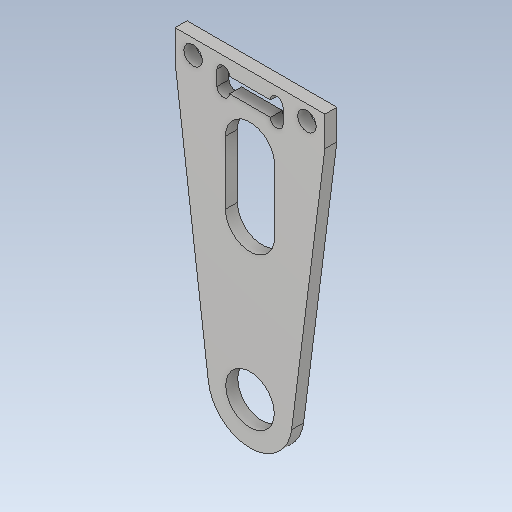
# Autodesk Inventor part: Leg_joint_slider_frame
Saved by Autodesk Inventor 2020.4 (Build 244396000, 396)
## iProperties
Part Number: Leg_joint_slider_frame
Material: アルミニウム 2014-T4
Document SubType Name: Modeling
Designer: Masato Kubotera
Density: 2.8 g/cm^3
Appearance: 滑らか - 淡い灰色
Mass: 4.69686 g
Surface Area: 22.2791 cm^2
Volume: 1.67745 cm^3
Description: A2017 T2
Author: Masato Kubotera
Autodesk Inventor part; units mm, degrees
ref_plane "YZ Plane" through (0, 0, 0) normal (1, 0, 0) x (0, 1, 0)
ref_plane "XZ Plane" through (0, 0, 0) normal (0, 1, 0) x (-1, 0, 0)
ref_plane "XY Plane" through (0, 0, 0) normal (0, 0, 1) x (1, 0, 0)
derived "Leg_joint_roll_basis.ipt"
sketch "スケッチ1" plane through (0, 0, 0) normal (0, 0, 1) x (1, 0, 0)
  circle A0 centre (0, 0) radius 11 construction
  line L0 (-13.5, -1) -> (13.5, -1) construction
  line L1 (13.5, -1) -> (13.5, -28) construction
  line L2 (13.5, -28) -> (-13.5, -28) construction
  line L3 (-13.5, -28) -> (-13.5, -1) construction
  line L4 (0, 18) -> (0, -18) construction
  circle A1 centre (0, -18) radius 7 construction
  line L5 (-12.5, 29.5) -> (-12.5, 24.5)
  line L6 (-12.5, 24.5) -> (-6.9433, -18.8892)
  line L7 (-12.5, 29.5) -> (12.5, 29.5)
  line L8 (12.5, 29.5) -> (12.5, 24.5)
  line L9 (12.5, 24.5) -> (6.9433, -18.8892)
  arc A2 (-6.9433, -18.8892) -> (6.9433, -18.8892) centre (0, -18) ccw
  circle A3 centre (-9.5, 27) radius 1.55
  circle A4 centre (9.5, 27) radius 1.55
  line L10 (-5.51, 27.01) -> (5.51, 27.01)
  line L11 (5.51, 27.01) -> (5.51, 24.49)
  line L12 (5.51, 24.49) -> (-5.51, 24.49)
  line L13 (-5.51, 24.49) -> (-5.51, 27.01)
  circle A5 centre (-4.46, 27.01) radius 1.05
  circle A6 centre (-4.46, 24.49) radius 1.05
  circle A7 centre (4.46, 27.01) radius 1.05
  circle A8 centre (4.46, 24.49) radius 1.05
  line L14 (5.5, 27) -> (-5.5, 27) construction
  line L15 (-5.5, 27) -> (-5.5, 24.5) construction
  line L16 (-5.5, 24.5) -> (5.5, 24.5) construction
  line L17 (5.5, 24.5) -> (5.5, 27) construction
  circle A9 centre (0, -18) radius 4.05
  circle A10 centre (0, 8.5) radius 1.35 construction
  circle A11 centre (-8.5, 0) radius 1.35 construction
  circle A12 centre (0, -8.5) radius 1.35 construction
  circle A13 centre (8.5, 0) radius 1.35 construction
  circle A14 centre (0, 0) radius 5.05 construction
  line L18 (-10.5671, 3.0556) -> (-5.7639, 19.6667) construction
  line L19 (5.7639, 19.6667) -> (10.5671, 3.0556) construction
  arc A15 (-10.5671, 3.0556) -> (10.5671, 3.0556) centre (0, 0) ccw construction
  arc A16 (5.7639, 19.6667) -> (-5.7639, 19.6667) centre (0, 18) ccw construction
  circle A17 centre (0, 18) radius 2.25 construction
  line L20 (-10.9105, 1.4) -> (-14.2125, 1.4) construction
  line L21 (-14.2125, 1.4) -> (-24.81, -5.5) construction
  line L22 (-24.81, -5.5) -> (-24.81, -23.5) construction
  line L23 (-24.81, -23.5) -> (-14.2125, -30.4) construction
  line L24 (-14.2125, -30.4) -> (14.2125, -30.4) construction
  line L25 (14.2125, -30.4) -> (24.81, -23.5) construction
  line L26 (24.81, -23.5) -> (24.81, -5.5) construction
  line L27 (24.81, -5.5) -> (14.2125, 1.4) construction
  line L28 (14.2125, 1.4) -> (10.9105, 1.4) construction
  arc A18 (-10.9105, 1.4) -> (10.9105, 1.4) centre (0, 0) ccw construction
  line L29 (-21.76, -10.49) -> (-19.74, -10.49) construction
  line L30 (-19.74, -10.49) -> (-19.74, -18.51) construction
  line L31 (-19.74, -18.51) -> (-21.76, -18.51) construction
  line L32 (-21.76, -18.51) -> (-21.76, -10.49) construction
  line L33 (-19.75, -10.5) -> (-21.75, -10.5) construction
  line L34 (-21.75, -10.5) -> (-21.75, -18.5) construction
  line L35 (-21.75, -18.5) -> (-19.75, -18.5) construction
  line L36 (-19.75, -18.5) -> (-19.75, -10.5) construction
  circle A19 centre (-21.76, -11.54) radius 1.05 construction
  circle A20 centre (-19.74, -11.54) radius 1.05 construction
  circle A21 centre (-19.74, -17.46) radius 1.05 construction
  circle A22 centre (-21.76, -17.46) radius 1.05 construction
  circle A23 centre (-13.5, -1) radius 2.4 construction
  line L37 (-24.81, -14.5) -> (-19.75, -14.5) construction
  circle A24 centre (-21.76, -11.54) radius 3.05 construction
  circle A25 centre (-13.5, -28) radius 2.4 construction
  line L38 (21.76, -10.49) -> (19.74, -10.49) construction
  line L39 (19.75, -10.5) -> (21.75, -10.5) construction
  circle A26 centre (19.74, -11.54) radius 1.05 construction
  circle A27 centre (21.76, -11.54) radius 1.05 construction
  circle A28 centre (21.76, -11.54) radius 3.05 construction
  line L40 (24.81, -14.5) -> (19.75, -14.5) construction
  line L41 (19.75, -18.5) -> (19.75, -10.5) construction
  line L42 (21.75, -10.5) -> (21.75, -18.5) construction
  line L43 (19.74, -10.49) -> (19.74, -18.51) construction
  line L44 (21.76, -18.51) -> (21.76, -10.49) construction
  circle A29 centre (19.74, -17.46) radius 1.05 construction
  line L45 (21.75, -18.5) -> (19.75, -18.5) construction
  line L46 (19.74, -18.51) -> (21.76, -18.51) construction
  circle A30 centre (21.76, -17.46) radius 1.05 construction
  line L47 (0, -14.813) -> (2.76, -16.4065) construction
  line L48 (2.76, -16.4065) -> (2.76, -19.5935) construction
  line L49 (2.76, -19.5935) -> (0, -21.187) construction
  line L50 (0, -21.187) -> (-2.76, -19.5935) construction
  line L51 (-2.76, -19.5935) -> (-2.76, -16.4065) construction
  line L52 (-2.76, -16.4065) -> (0, -14.813) construction
  line L53 (-19.75, 12) -> (19.75, 12) construction
  line L54 (19.75, 12) -> (19.75, -39.5) construction
  line L55 (19.75, -39.5) -> (-19.75, -39.5) construction
  line L56 (-19.75, -39.5) -> (-19.75, 12) construction
  arc A31 (4.1, 18) -> (-4.1, 18) centre (0, 18) ccw
  line L57 (-4.1, 18) -> (-4.1, 7.4558)
  line L58 (4.1, 18) -> (4.1, 7.4558)
  arc A32 (-4.1, 7.4558) -> (4.1, 7.4558) centre (0, 7.4558) ccw
  circle A33 centre (0, 18) radius 6.5 construction
  line L59 (-21.75, -2) -> (-19.75, -2) construction
  line L60 (-19.75, -2) -> (-19.75, -27) construction
  line L61 (-19.75, -27) -> (-21.75, -27) construction
  line L62 (-21.75, -27) -> (-21.75, -2) construction
  circle A34 centre (0, -18) radius 36 construction
  line L63 (0, -18) -> (-25.4558, 7.4558) construction
  circle A35 centre (0, 0) radius 18 construction
  line L64 (-18, 0) -> (-25.4558, 7.4558) construction
  circle A36 centre (0, -18) radius 1.55
  circle A37 centre (-13.5, -28) radius 1.35
  arc A38 (-13.5, 0.35) -> (-13.5, -2.35) centre (-13.5, -1) ccw
  arc A39 (-12.5, -2.35) -> (-12.5, 0.35) centre (-12.5, -1) ccw
  line L65 (-12.5, 0.35) -> (-13.5, 0.35)
  line L66 (-13.5, -2.35) -> (-12.5, -2.35)
  line L67 (13.5, -2.35) -> (12.5, -2.35)
  arc A40 (13.5, -2.35) -> (13.5, 0.35) centre (13.5, -1) ccw
  line L68 (12.5, 0.35) -> (13.5, 0.35)
  arc A41 (12.5, 0.35) -> (12.5, -2.35) centre (12.5, -1) ccw
  circle A42 centre (13.5, -28) radius 1.35
  arc A43 (0.9093, -15.338) -> (-0.9093, -15.338) centre (0, -15.863) ccw construction
  arc A44 (-1.8507, -15.8815) -> (-2.76, -17.4565) centre (-1.8507, -16.9315) ccw construction
  arc A45 (-2.76, -18.5435) -> (-1.8507, -20.1185) centre (-1.8507, -19.0685) ccw construction
  arc A46 (-0.9093, -20.662) -> (0.9093, -20.662) centre (0, -20.137) ccw construction
  arc A47 (1.8507, -20.1185) -> (2.76, -18.5435) centre (1.8507, -19.0685) ccw construction
  arc A48 (2.76, -17.4565) -> (1.8507, -15.8815) centre (1.8507, -16.9315) ccw construction
  line L69 (-1.8507, -15.8815) -> (-0.9093, -15.338) construction
  line L70 (0.9093, -15.338) -> (1.8507, -15.8815) construction
  line L71 (2.76, -17.4565) -> (2.76, -18.5435) construction
  line L72 (1.8507, -20.1185) -> (0.9093, -20.662) construction
  line L73 (-0.9093, -20.662) -> (-1.8507, -20.1185) construction
  line L74 (-2.76, -18.5435) -> (-2.76, -17.4565) construction
  circle A49 centre (0, 0) radius 10.5 construction
  line L75 (-10.9105, 1.4) -> (10.9105, 1.4)
  arc A50 (-10.6584, 1.4) -> (10.6557, 1.4208) centre (0, 0) ccw
  circle A51 centre (0, -18) radius 3
  circle A52 centre (0, -18) radius 2.25
  point P0 (0, -1)
  point P1 (0, 29.5)
  point P2 (-12.5, 27)
  point P3 (-21.75, -14.5)
  point P4 (-2.76, -16.4065)
  point P5 (-2.76, -19.5935)
  point P6 (2.76, -19.5935)
  point P7 (2.76, -16.4065)
extrude "押し出し1" add sketch "スケッチ1" along normal blind 2 contours L7 L8 L9 L75 L6 L5 | L75 L9 A50 L6 | A50 L9 A2 L6
